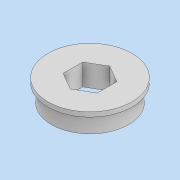
# Autodesk Inventor part: Bearing
Saved by Autodesk Inventor 2022 (Build 260153000, 153)
## iProperties
Created: 2023-02-11
Part Number: Bearing
Material: Generic
Document SubType Name: Modeling
Designer: coled
Density: 1 g/cm^3
Appearance: Default
Author: coled
Autodesk Inventor part; units mm, degrees
ref_plane "YZ Plane" through (0, 0, 0) normal (1, 0, 0) x (0, 1, 0)
ref_plane "XZ Plane" through (0, 0, 0) normal (0, 1, 0) x (-1, 0, 0)
ref_plane "XY Plane" through (0, 0, 0) normal (0, 0, 1) x (1, 0, 0)
sketch "Sketch1" plane through (0, 0, 0) normal (0, 1, 0) x (-1, 0, 0)
  circle A0 centre (0, 0) radius 14.31
  line L0 (0, 0) -> (6.335, 0)
  line L1 (6.335, -3.6575) -> (0, -7.315)
  line L2 (0, -7.315) -> (-6.335, -3.6575)
  line L3 (-6.335, -3.6575) -> (-6.335, 3.6575)
  line L4 (-6.335, 3.6575) -> (0, 7.315)
  line L5 (0, 7.315) -> (6.335, 3.6575)
  line L6 (6.335, 3.6575) -> (6.335, -3.6575)
  dimension "d0" = 28.62
  dimension "d1" = 6.335
  constraints: 14 end point, 2 coincident, 1 centre point, 1 horizontal, 1 midpoint, 13 other
  measures "d0" diameter of A0
  measures "d1" distance of L0.start L0.end
extrude "Extrusion1" add sketch "Sketch1" along normal blind 8
sketch "Sketch2" plane through (0, 8, 0) normal (0, 1, 0) x (1, 0, 0)
  circle A0 centre (0, 0) radius 15.585
  line L0 (-6.335, -3.6575) -> (-6.335, 3.6575) projected
  line L1 (-6.335, 3.6575) -> (0, 7.315)
  line L2 (0, 7.315) -> (6.335, 3.6575)
  line L3 (6.335, 3.6575) -> (6.335, -3.6575)
  line L4 (6.335, -3.6575) -> (0, -7.315)
  line L5 (0, -7.315) -> (-6.335, -3.6575)
  line L6 (-6.335, -3.6575) -> (-6.335, 3.6575)
  point P0 (-6.335, 0)
  dimension "d4" = 31.17
  constraints: 12 end point, 2 coincident, 2 midpoint, 1 centre point, 13 other
  measures "d4" diameter of A0
extrude "Extrusion2" add sketch "Sketch2" against normal blind 1.7
body "Solid1"
